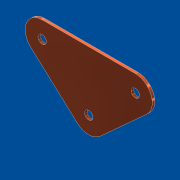
# Autodesk Inventor part: Conexion_eje
Saved by Autodesk Inventor 2016 (Build 200138000, 138)
## iProperties
Created: 2017-05-13
Part Number: Conexion_eje
Material: Generic
Document SubType Name: Sheet Metal
Designer: Gian
Density: 1 g/cm^3
Sheet Metal Rule: Default_mm
Appearance: Default
Author: Gian
Autodesk Inventor part; units mm, degrees
ref_plane "YZ Plane" through (0, 0, 0) normal (1, 0, 0) x (0, 1, 0)
ref_plane "XZ Plane" through (0, 0, 0) normal (0, 1, 0) x (-1, 0, 0)
ref_plane "XY Plane" through (0, 0, 0) normal (0, 0, 1) x (1, 0, 0)
sketch "Sketch1" plane through (0, 0, 0) normal (0, 1, 0) x (-1, 0, 0)
  line L0 (6.5166, 8.4883) -> (-103.4834, 8.4883) construction
  circle A0 centre (6.5166, 8.4883) radius 5
  circle A1 centre (-103.4834, 8.4883) radius 5
  line L1 (-48.4834, 8.4883) -> (-48.4834, -41.5117) construction
  circle A2 centre (-48.4834, -41.5117) radius 5
  line L2 (6.5166, 13.4883) -> (6.5166, 28.4883) construction
  arc A3 (20.6341, -5.6784) -> (6.5166, 28.4883) centre (6.5166, 8.4883) ccw
  arc A4 (-103.4834, 28.4883) -> (-116.9369, -6.3105) centre (-103.4834, 8.4883) ccw
  arc A5 (-61.9369, -56.3105) -> (-35.0258, -56.3068) centre (-48.4834, -41.5117) ccw
  line L3 (20.6341, -5.6784) -> (-35.0258, -56.3068)
  line L4 (6.5166, 28.4883) -> (-103.4834, 28.4883)
  line L5 (-116.9369, -6.3105) -> (-61.9369, -56.3105)
  line L6 (-48.4834, -36.5117) -> (-48.4834, -16.5117)
  dimension "d1" = 10
  dimension "d4" = 10
  dimension "d0" = 110
  dimension "d2" = 10
  dimension "d3" = 50
  dimension "d5" = 15
  dimension "d6" = 15
  dimension "d7" = 15
  dimension "d12" = 20
  measures "d0" distance of L0.start L0.end
  measures "d2" diameter of A1
  measures "d3" distance of L1.start L1.end
  measures "d5" distance of L2.end L2.start
  measures "d6" radial gap between concentric circles of A1 A4
  measures "d12" distance of L6.start L6.end
extrude "Plate1" add sketch "Sketch1" along normal blind 3
equation "\"BendRadius\" = Thickness"
equation "\"BendReliefWidth\" = Thickness"
equation "\"BendReliefDepth\" = 0.5 * Thickness"
equation "\"CornerReliefSize\" = 4 * Thickness"
equation "\"MinimumRemnant\" = 2 * Thickness"
equation "\"TransitionRadius\" = BendRadius"
equation "\"JacobiRadiusSize\" = BendRadius"
equation "\"GapSize\" = Thickness"
equation "\"d8\" = BendRadius"
equation "\"Thickness\" = 3"
body "Solid1"
